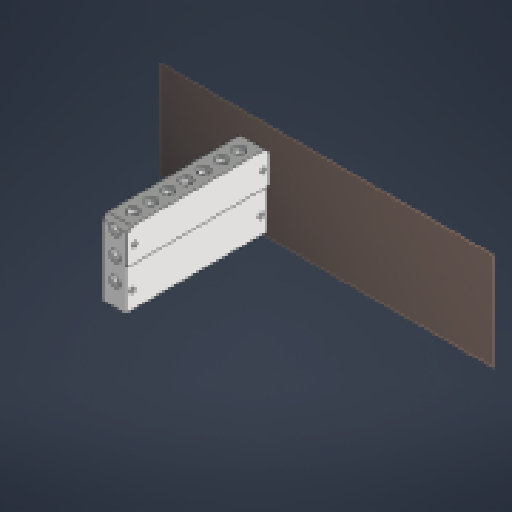
# Autodesk Inventor part: stepper motor controller mount
Saved by Autodesk Inventor 2026.3 (Build 303398000, 398)
## iProperties
Created: 2026-04-19
Part Number: stepper motor controller mount
Material: Generic
Document SubType Name: Modeling
Designer: micha
Density: 1 g/cm^3
Appearance: Default
Author: micha
Autodesk Inventor part; units mm, degrees
ref_plane "YZ Plane" through (0, 0, 0) normal (1, 0, 0) x (0, 1, 0)
ref_plane "XZ Plane" through (0, 0, 0) normal (0, 1, 0) x (-1, 0, 0)
ref_plane "XY Plane" through (0, 0, 0) normal (0, 0, 1) x (1, 0, 0)
ref_plane "Work Plane1" through (0, 0, 0) normal (0, 0, 1) x (1, 0, 0)
sketch "Sketch1" plane through (0, 0, 0) normal (0, 0, 1) x (1, 0, 0)
  line L0 (-40.3123, -16.219) -> (-40.3123, -1.919) projected
  line L1 (-38.8123, 20.681) -> (-36.2123, 20.681) projected
  line L2 (-38.8123, 20.681) -> (-38.8123, 11.381) projected
  line L3 (-38.8123, 6.881) -> (-38.8123, -7.419) projected
  line L4 (-38.8123, 11.381) -> (-38.8123, 6.881) projected
  line L5 (-55.7184, -30.019) -> (-40.3123, -30.019)
  line L6 (-40.3123, -30.019) -> (-40.3123, -1.919)
  line L7 (-40.3123, -1.919) -> (-55.7184, -1.919)
  line L8 (-55.7184, -1.919) -> (-55.7184, -30.019)
  line L9 (-55.7184, -1.919) -> (-38.8123, -1.919)
  line L10 (-38.8123, -1.919) -> (-38.8123, 20.681)
  line L11 (-38.8123, 20.681) -> (-55.7184, 20.681)
  line L12 (-55.7184, 20.681) -> (-55.7184, -1.919)
  circle A0 centre (-17.481, -14.981) radius 3 projected
  circle A1 centre (-17.481, 0.019) radius 3 projected
  circle A2 centre (-17.481, 15.019) radius 3 projected
  circle A3 centre (-17.481, 15.019) radius 2.65
  circle A4 centre (-17.481, -14.981) radius 2.65
  circle A5 centre (-17.481, 0.019) radius 2.65
  point P0 (0, 0)
  point P1 (-40.3123, -30.019)
  dimension "d9" = 6
  dimension "d10" = 5.3
  dimension "d11" = 5.3
  dimension "d12" = 5.3
  constraints: 16 end point, 4 parallel, 3 centre point, 3 coincident, 2 horizontal, 2 perpendicular, 2 other
  measures "d9" diameter of A2
  measures "d10" diameter of A3
  measures "d11" diameter of A4
  measures "d12" diameter of A5
extrude "Extrusion1" add sketch "Sketch1" along normal blind 96
sketch "Sketch2" plane through (-38.8123, -1.919, 0) normal (1, 0, 0) x (0, 0, -1)
  arc A0 (-4.35, 13.3) -> (-4.35, 8.8) centre (-4.35, 11.05) ccw projected
  arc A1 (-4.35, -14.3) -> (-4.35, -18.8) centre (-4.35, -16.55) ccw projected
  circle A2 centre (-4.35, 11.05) radius 1.75
  circle A3 centre (-4.35, -16.55) radius 1.75
  line L0 (-96, 22.6) -> (-96, -28.1) projected
  line L1 (0, 22.6) -> (0, -28.1) projected
  line L2 (-96, 22.6) -> (0, 22.6)
  line L3 (0, 22.6) -> (-48, 22.6)
  line L4 (-48, -36.2747) -> (-48, 22.6)
  circle A4 centre (-91.65, 11.05) radius 1.75
  circle A5 centre (-91.65, -16.55) radius 1.75
  point P0 (0, 1.919)
  dimension "d2" = 3.5
  dimension "d3" = 3.5
  constraints: 6 end point, 4 centre point, 2 coincident, 2 symmetric about line, 1 horizontal, 1 midpoint, 1 perpendicular, 2 other
  measures "d2" diameter of A2
  measures "d3" diameter of A3
extrude "Extrusion2" cut sketch "Sketch2" against normal through all
chamfer "Chamfer1" distance 3 angle 45 2 edges at (-47.2653, 20.681, 0) (-47.2653, 20.681, 96)
sketch "Sketch3" plane through (-55.7184, 20.681, 93) normal (0, 1, 0) x (1, 0, 0)
  line L0 (0, -3) -> (16.9061, -3) projected
  line L1 (16.9061, -3) -> (0, -3)
  line L2 (8.453, -3) -> (8.453, 93)
  circle A0 centre (8.453, 9) radius 2.75
  line L3 (0, -3) -> (0, 93)
  line L4 (0, 93) -> (0, 45)
  line L5 (0, 90) -> (0, 0) projected
  line L6 (15.4061, 93) -> (15.4061, -3) projected
  line L7 (15.4061, 45) -> (0, 45)
  line L8 (35.5874, -3) -> (35.5874, 93) projected
  circle A1 centre (8.453, 21) radius 2.75
  circle A2 centre (8.453, 33) radius 2.75
  circle A3 centre (8.453, 45) radius 2.75
  line L9 (16.9061, 0) -> (0, 0) projected
  circle A4 centre (8.453, 81) radius 2.75
  circle A5 centre (8.453, 69) radius 2.75
  circle A6 centre (8.453, 57) radius 2.75
  point P0 (55.7184, 93)
  dimension "d13" = 5.5
  dimension "d14" = 12
  dimension "d15" = 5.5
  dimension "d16" = 12
  dimension "d17" = 5.5
  dimension "d18" = 12
  dimension "d19" = 5.5
  dimension "d20" = 45
  dimension "d21" = 48
  dimension "d22" = 12
  dimension "d23" = 12
  constraints: 10 end point, 7 centre point, 5 midpoint, 4 point on line, 3 symmetric about line, 2 vertical, 1 collinear, 1 perpendicular, 3 other
  measures "d13" diameter of A0
  measures "d14" distance from line of L0 A0.centre
  measures "d15" diameter of A1
  measures "d16" distance of A1.centre A0.centre
  measures "d17" diameter of A2
  measures "d18" distance of A2.centre A1.centre
  measures "d19" diameter of A3
  measures "d20" distance between parallel lines of L7 L9
  measures "d21" distance between parallel lines of L0 L7
  measures "d22" distance of A3.centre A2.centre
  measures "d23" distance of point (8.453, 45) A2.centre
extrude "Extrusion3" cut sketch "Sketch3" against normal through all contours A0 L2 | L2 A0 | A3 L2 L7 | L7 L2 A3 | L7 A3 L2 | L2 A3 L7 | A1 L2 | L2 A1 | A2 L2 | L2 A2 | A6 L2 | L2 A6 | A5 L2 | L2 A5 | A4 L2 | L2 A4
chamfer "Chamfer2" [suppressed]
body "Solid1"
